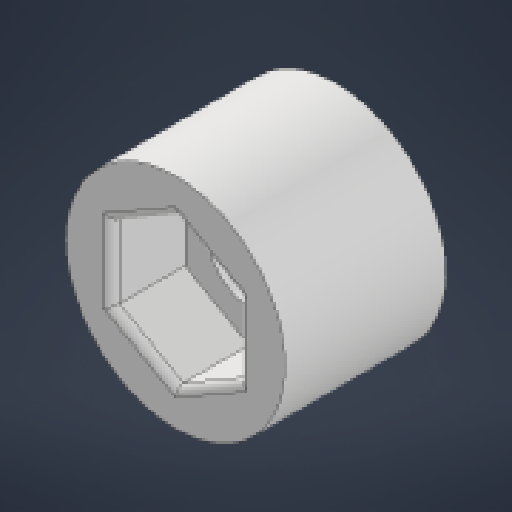
# Autodesk Inventor part: ActuatorSpacer
Saved by Autodesk Inventor 2026.2 (Build 302298000, 298)
## iProperties
Created: 2026-03-15
Part Number: ActuatorSpacer
Material: Generic
Document SubType Name: Modeling
Designer: brand
Density: 1 g/cm^3
Appearance: Default
Author: brand
Autodesk Inventor part; units mm, degrees
ref_plane "YZ Plane" through (0, 0, 0) normal (1, 0, 0) x (0, 1, 0)
ref_plane "XZ Plane" through (0, 0, 0) normal (0, 1, 0) x (-1, 0, 0)
ref_plane "XY Plane" through (0, 0, 0) normal (0, 0, 1) x (1, 0, 0)
sketch "Sketch1" plane through (0, 0, 0) normal (0, 0, 1) x (1, 0, 0)
  circle A0 centre (109.5845, 54.716) radius 3.175 construction
  line L0 (765.556, 95.25) -> (765.556, -44.45) construction
  line L1 (0, 95.25) -> (765.556, 95.25) construction
  line L2 (0, -44.45) -> (0, 95.25) construction
  line L3 (765.556, -44.45) -> (0, -44.45) construction
  arc A1 (100.6141, 53.9869) -> (110.3117, 45.7454) centre (109.5836, 54.7149) ccw projected
  line L4 (123.1622, 19.6987) -> (119.3655, 66.4721) projected
  circle A2 centre (109.5836, 54.7149) radius 8.999
  circle A3 centre (109.5845, 54.716) radius 6 projected
  circle A4 centre (109.5845, 54.716) radius 6.254
  circle A5 centre (109.5845, 54.716) radius 3.3
  point P0 (0, 0)
  dimension "d0" = 0.254
  dimension "d1" = 6.6
  constraints: 2 centre point, 2 coincident, 3 other
  measures "d0" radial gap between concentric circles of A3 A4
  measures "d1" diameter of A5
extrude "Extrusion1" add sketch "Sketch1" along normal blind 7.1882 contours A2 A1 | A3 | A4
sketch "Sketch2" plane through (109.5836, 54.7149, 7.1882) normal (0, 0, 1) x (1, 0, 0)
  circle A0 centre (0.0009, 0.0011) radius 3.3 projected
  line L0 (-4.9991, 2.8878) -> (0.0009, 5.7746)
  line L1 (0.0009, 5.7746) -> (5.0009, 2.8878)
  line L2 (5.0009, 2.8878) -> (5.0009, -2.8857)
  line L3 (5.0009, -2.8857) -> (0.0009, -5.7724)
  line L4 (0.0009, -5.7724) -> (-4.9991, -2.8857)
  line L5 (-4.9991, -2.8857) -> (-4.9991, 2.8878)
  line L6 (0.0009, 6.0679) -> (-5.2531, 3.0345)
  line L7 (-5.2531, 3.0345) -> (-5.2531, -3.0323)
  line L8 (-5.2531, -3.0323) -> (0.0009, -6.0657)
  line L9 (0.0009, -6.0657) -> (5.2549, -3.0323)
  line L10 (5.2549, -3.0323) -> (5.2549, 3.0345)
  line L11 (5.2549, 3.0345) -> (0.0009, 6.0679)
  circle A1 centre (0, 0) radius 8.999 projected
  point P0 (-109.5836, -54.7149)
  point P1 (-4.9991, -2.8857)
  dimension "d4" = 0.254
  constraints: 24 end point, 1 coincident, 20 other
  measures "d4" distance between parallel lines of L0 L6
extrude "Extrusion2" add sketch "Sketch2" along normal blind 6.0198 contours A1
fillet "Fillet1" radius 0.635 6 edges at (104.3305, 54.716, 13.208) (106.9575, 50.1659, 13.208) (112.2115, 50.1659, 13.208) (114.8385, 54.716, 13.208) (112.2115, 59.2661, 13.208) (106.9575, 59.2661, 13.208)
body "Solid1"
